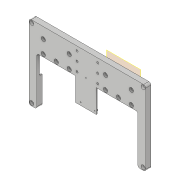
# Autodesk Inventor part: 10_Baseplate
Saved by Autodesk Inventor 2019 (Build 230136000, 136)
## iProperties
Created: 2019-05-14
Part Number: 10_Baseplate
Material: Generic
Document SubType Name: Modeling
Designer: diederichbenedict
Density: 1 g/cm^3
Appearance: Default
Author: diederichbenedict
Autodesk Inventor part; units mm, degrees
ref_plane "YZ Plane" through (0, 0, 0) normal (1, 0, 0) x (0, 1, 0)
ref_plane "XZ Plane" through (0, 0, 0) normal (0, 1, 0) x (-1, 0, 0)
ref_plane "XY Plane" through (0, 0, 0) normal (0, 0, 1) x (1, 0, 0)
ref_plane "Work Plane1" through (0, 0, 0) normal (0, 0, 1) x (1, 0, 0)
sketch "Sketch1" plane through (0, 0, 0) normal (0, 0, 1) x (1, 0, 0)
  circle A0 centre (0, 25) radius 1.95 construction
  circle A1 centre (-25, 0) radius 1.95 projected
  circle A2 centre (-25, -25) radius 1.95 projected
  circle A3 centre (25, 25) radius 1.95 construction
  circle A4 centre (25, -25) radius 1.95 projected
  circle A5 centre (-25, 25) radius 1.95 construction
  circle A6 centre (25, 0) radius 1.95 projected
  circle A7 centre (0, -25) radius 1.95 projected
  line L0 (-28, 30) -> (-30, 28) construction
  line L1 (-30, 28) -> (-30, -28) construction
  line L2 (-30, -28) -> (-28, -30) construction
  line L3 (-28, -30) -> (28, -30) construction
  line L4 (28, -30) -> (30, -28) construction
  line L5 (30, -28) -> (30, 28) construction
  line L6 (30, 28) -> (28, 30) construction
  line L7 (28, 30) -> (-28, 30) construction
  circle A8 centre (-145, 0) radius 1.95 projected
  circle A9 centre (-120, -25) radius 1.95 projected
  circle A10 centre (-95, -25) radius 1.95 projected
  circle A11 centre (-145, 25) radius 1.95 construction
  circle A12 centre (-95, 25) radius 1.95 construction
  circle A13 centre (-145, -25) radius 1.95 projected
  circle A14 centre (-120, 25) radius 1.95 construction
  circle A15 centre (-95, 0) radius 1.95 projected
  line L8 (-150, -28) -> (-148, -30) construction
  line L9 (-148, -30) -> (-92, -30) construction
  line L10 (-92, -30) -> (-90, -28) construction
  line L11 (-90, -28) -> (-90, 28) construction
  line L12 (-90, 28) -> (-92, 30) construction
  line L13 (-92, 30) -> (-148, 30) construction
  line L14 (-148, 30) -> (-150, 28) construction
  line L15 (-150, 28) -> (-150, -28) construction
  circle A16 centre (-167.5, -118) radius 1.95 projected
  circle A17 centre (47.5, -118) radius 1.95 construction
  circle A18 centre (47.5, 16) radius 1.95 projected
  circle A19 centre (-167.5, 16) radius 1.95 projected
  line L16 (52.5, -123) -> (-172.5, -123) construction
  line L17 (-172.5, -123) -> (-172.5, 21) construction
  line L18 (-172.5, 21) -> (52.5, 21) construction
  line L19 (52.5, 21) -> (52.5, -123) construction
  line L20 (52.5, -123) -> (37.5, -123) construction
  line L21 (37.5, -123) -> (37.5, 21) construction
  line L22 (37.5, 21) -> (52.5, 21) construction
  line L23 (52.5, 21) -> (52.5, -123) construction
  line L24 (-172.5, -123) -> (-157.5, -123) construction
  line L25 (-157.5, -123) -> (-157.5, 21) construction
  line L26 (-157.5, 21) -> (-172.5, 21) construction
  line L27 (-172.5, 21) -> (-172.5, -123) construction
  line L28 (-30, -30) -> (37.5, -30) construction
  line L29 (37.5, -30) -> (37.5, 21) construction
  line L30 (37.5, 21) -> (-30, 21) construction
  line L31 (-30, 21) -> (-30, -30) construction
  line L32 (-157.5, 21) -> (-90, 21) construction
  line L33 (-90, 21) -> (-90, -30) construction
  line L34 (-90, -30) -> (-157.5, -30) construction
  line L35 (-157.5, -30) -> (-157.5, 21) construction
  circle A20 centre (47.5, -118) radius 1.95
  line L36 (52.5, 21) -> (-172.5, 21)
  line L37 (-172.5, 21) -> (-172.5, -30)
  line L38 (-172.5, -30) -> (52.5, -30)
  line L39 (52.5, -30) -> (52.5, 21)
  line L40 (-172.5, -123) -> (-157.5, -123)
  line L41 (-157.5, -123) -> (-157.5, -30)
  line L42 (-157.5, -30) -> (-172.5, -30)
  line L43 (-172.5, -30) -> (-172.5, -123)
  line L44 (52.5, -123) -> (37.5, -123)
  line L45 (37.5, -123) -> (37.5, -30)
  line L46 (37.5, -30) -> (52.5, -30)
  line L47 (52.5, -30) -> (52.5, -123)
  line L48 (-80, 13) -> (-40, 13) construction
  line L49 (-40, 13) -> (-40, -22) construction
  line L50 (-40, -22) -> (-80, -22) construction
  line L51 (-80, -22) -> (-80, 13) construction
  line L52 (-80, 13) -> (-40, -22) construction
  line L53 (-40, 13) -> (-80, -22) construction
  circle A21 centre (-80, -4.5) radius 1.95
  circle A22 centre (-80, 13) radius 1.95
  circle A23 centre (-80, -22) radius 1.95
  circle A24 centre (-40, -22) radius 1.95
  circle A25 centre (-40, 13) radius 1.95
  circle A26 centre (-40, -4.5) radius 1.95
  point P0 (0, 0)
  point P1 (-60, -4.5)
  dimension "d0" = 5
  dimension "d1" = 5
  dimension "d2" = 5
  dimension "d3" = 5
  dimension "d4" = 15
  dimension "d5" = 15
  dimension "d33" = 40
  dimension "d34" = 35
  dimension "d35" = 17.5
  dimension "d36" = 17.5
  dimension "d37" = 3.9
  dimension "d38" = 3.9
  dimension "d39" = 3.9
  dimension "d40" = 3.9
  dimension "d41" = 3.9
  dimension "d42" = 3.9
  constraints: 76 end point, 18 parallel, 9 horizontal, 9 perpendicular, 7 centre point, 7 coincident, 4 midpoint, 4 point on line, 1 concentric
  measures "d0" distance from line of L19 A17.centre
  measures "d1" distance from line of A17.centre L16
  measures "d2" distance from line of A16.centre L17
  measures "d3" distance from line of A19.centre L18
  measures "d4" distance of L21.end L22.end
  measures "d5" distance of L26.end L25.end
  measures "d33" distance of L49.end L50.end
  measures "d34" distance of L48.end L49.end
  measures "d35" distance from line of point (-80, -4.5) L50
  measures "d36" distance from line of L50 point (-40, -4.5)
  measures "d37" diameter of A21
  measures "d38" diameter of A22
  measures "d39" diameter of A23
  measures "d40" diameter of A24
  measures "d41" diameter of A25
  measures "d42" diameter of A26
extrude "Extrusion1" add sketch "Sketch1" along normal blind 10
ref_plane "Work Plane2" through (-76.1, -69.7723, 8.1376) normal (0, -1, 0) x (-1, 0, 0)
ref_plane "Work Plane3" through (-64.05, -74.8223, 4.8376) normal (0, 1, 0) x (0, 0, 1)
sketch "Sketch2" plane through (-76.1, -69.7723, 8.1376) normal (0, -1, 0) x (-1, 0, 0)
  line L0 (6.9, 4.3) -> (-1.2981, 4.3) construction
  line L1 (-1.2981, 4.3) -> (-1.2981, 3.3) construction
  line L2 (-1.2981, 3.3) -> (0, 3.3) construction
  line L3 (0, 2.5) -> (0, 3.3) construction
  line L4 (0, 2.5) -> (-1.65, 2.5) construction
  line L5 (-1.65, 0) -> (-1.65, 2.5) construction
  line L6 (6.9, 0) -> (-1.65, 0) construction
  line L7 (6.9, 0) -> (6.9, 4.3) construction
  line L8 (-32.1, 2.3) -> (-32.1, 4.3) construction
  line L9 (-32.1, 4.3) -> (-33.3, 4.3) construction
  line L10 (-33.3, 0) -> (-33.3, 4.3) construction
  line L11 (-33.3, 0) -> (-28.35, 0) construction
  line L12 (-28.35, 0) -> (-28.35, 2.3) construction
  line L13 (-28.35, 2.3) -> (-32.1, 2.3) construction
  line L14 (81.4, -1.8624) -> (-113.6, -1.8624) construction
  line L15 (-33.3, 0) -> (6.9, 0)
  line L16 (6.9, 0) -> (6.9, -1.8624)
  line L17 (6.9, -1.8624) -> (-33.3, -1.8624)
  line L18 (-33.3, -1.8624) -> (-33.3, 0)
  point P0 (-76.1, 8.1376)
  constraints: 8 end point, 2 parallel, 1 horizontal, 1 perpendicular, 1 point on line
extrude "Extrusion2" add sketch "Sketch2" along normal up to surface (44.8223 mm away) from surface at -39.7723
sketch "Sketch3" plane through (-42.8, -69.7723, 8.1376) normal (0, 0, -1) x (-1, 0, 0)
  line L0 (0, 39.7723) -> (40.2, 39.7723) projected
  line L1 (0, 39.7723) -> (0, -5.05) projected
  line L2 (40.2, -5.05) -> (40.2, 39.7723) projected
  line L3 (114.7, 39.7723) -> (40.2, 39.7723) projected
  arc A0 (40.2, 39.7723) -> (0, 39.7723) centre (20.1, 30.1966) ccw
  line L4 (40.2, -5.05) -> (0, -5.05) projected
  point P0 (-42.8, 69.7723)
  constraints: 2 point on circle, 1 centre point
extrude "Extrusion3" cut sketch "Sketch3" along normal up to surface (8.1376 mm away) contours A0 L0
sketch "Sketch4" plane through (-42.8, -74.8223, 8.1376) normal (0, 0, -1) x (-1, 0, 0)
  circle A0 centre (3.3, 4.4309) radius 0.9 projected
  circle A1 centre (20, 51.15) radius 0.9 projected
  circle A2 centre (30.3, 5.3) radius 0.9 projected
  point P0 (-42.8, 74.8223)
extrude "Extrusion4" cut sketch "Sketch4" against normal through all
sketch "Sketch5" plane through (-42.8, -74.8223, 8.1376) normal (0, 0, -1) x (-1, 0, 0)
  circle A0 centre (20, 51.15) radius 0.9 projected
  circle A1 centre (3.3, 4.4309) radius 0.9 projected
  circle A2 centre (30.3, 5.3) radius 0.9 projected
  circle A3 centre (20, 51.15) radius 2.1
  circle A4 centre (3.3, 4.4309) radius 2.1
  circle A5 centre (30.3, 5.3) radius 2.1
  point P0 (-42.8, 74.8223)
  dimension "d14" = 1.2
  dimension "d15" = 1.2
  dimension "d16" = 1.2
  constraints: 3 centre point
  measures "d14" radial gap between concentric circles of A0 A3
  measures "d15" radial gap between concentric circles of A1 A4
  measures "d16" radial gap between concentric circles of A2 A5
ref_plane "Work Plane4" through (-51.8, -75.6302, 5.8376) normal (0, 0, 1) x (1, 0, 0)
extrude "Extrusion5" add sketch "Sketch5" along normal up to surface (2.3 mm away)
sketch "Sketch6" plane through (-62.8, -23.6723, 5.8376) normal (0, 0, -1) x (-1, 0, 0)
  circle A0 centre (0, 0) radius 2.1 projected
  circle A1 centre (0, 0) radius 0.9 projected
  point P0 (-62.8, 23.6723)
ref_plane "Work Plane5" through (-72.8, -36.4723, 4.6376) normal (0, 0, 1) x (1, 0, 0)
extrude "Extrusion6" add sketch "Sketch6" along normal up to surface (1.2 mm away)
fillet "Fillet1" radius 4 8 edges at (37.5, -123, 5) (52.5, -123, 5) (37.5, -30, 5) (-172.5, -123, 5) (-157.5, -123, 5) (-157.5, -30, 5) (-172.5, 21, 5) (52.5, 21, 5)
sketch "Sketch7" plane through (0, 0, 10) normal (0, 0, 1) x (1, 0, 0)
  arc A0 (52.5, 17) -> (48.5, 21) centre (48.5, 17) ccw projected
  line L0 (48.5, 21) -> (-168.5, 21) projected
  arc A1 (-168.5, 21) -> (-172.5, 17) centre (-168.5, 17) ccw projected
  line L1 (-172.5, 17) -> (-172.5, -119) projected
  arc A2 (-172.5, -119) -> (-168.5, -123) centre (-168.5, -119) ccw projected
  line L2 (-168.5, -123) -> (-161.5, -123) projected
  arc A3 (-161.5, -123) -> (-157.5, -119) centre (-161.5, -119) ccw projected
  line L3 (-157.5, -119) -> (-157.5, -34) projected
  arc A4 (-153.5, -30) -> (-157.5, -34) centre (-153.5, -34) ccw projected
  line L4 (-153.5, -30) -> (-83, -30) projected
  line L5 (-83, -74.8223) -> (-83, -30) projected
  line L6 (-42.8, -74.8223) -> (-83, -74.8223) projected
  line L7 (-42.8, -74.8223) -> (-42.8, -30) projected
  line L8 (-42.8, -30) -> (33.5, -30) projected
  arc A5 (37.5, -34) -> (33.5, -30) centre (33.5, -34) ccw projected
  line L9 (37.5, -34) -> (37.5, -119) projected
  arc A6 (37.5, -119) -> (41.5, -123) centre (41.5, -119) ccw projected
  line L10 (41.5, -123) -> (48.5, -123) projected
  arc A7 (48.5, -123) -> (52.5, -119) centre (48.5, -119) ccw projected
  line L11 (52.5, -119) -> (52.5, 17) projected
  circle A8 centre (-62.8, -23.6723) radius 0.9 projected
  circle A9 centre (-46.1, -70.3914) radius 0.9 projected
  circle A10 centre (-73.1, -69.5223) radius 0.9 projected
  circle A11 centre (-167.5, 16) radius 1.95 projected
  circle A12 centre (47.5, 16) radius 1.95 projected
  circle A13 centre (-95, 0) radius 1.95 projected
  circle A14 centre (-145, -25) radius 1.95 projected
  circle A15 centre (-95, -25) radius 1.95 projected
  circle A16 centre (-120, -25) radius 1.95 projected
  circle A17 centre (-145, 0) radius 1.95 projected
  circle A18 centre (0, -25) radius 1.95 projected
  circle A19 centre (25, 0) radius 1.95 projected
  circle A20 centre (25, -25) radius 1.95 projected
  circle A21 centre (-25, -25) radius 1.95 projected
  circle A22 centre (-25, 0) radius 1.95 projected
  circle A23 centre (-167.5, -118) radius 1.95 projected
  circle A24 centre (47.5, -118) radius 1.95 projected
  circle A25 centre (-40, -4.5) radius 1.95 projected
  circle A26 centre (-40, 13) radius 1.95 projected
  circle A27 centre (-40, 13) radius 1.95 projected
  circle A28 centre (-40, -22) radius 1.95 projected
  circle A29 centre (-40, -22) radius 1.95 projected
  circle A30 centre (-80, -22) radius 1.95 projected
  circle A31 centre (-80, -4.5) radius 1.95 projected
  circle A32 centre (-80, -4.5) radius 1.95 projected
  circle A33 centre (-80, 13) radius 1.95 projected
  circle A34 centre (-80, 13) radius 1.95 projected
  point P0 (0, 0)
hole "Hole1" at (47.5, 16, 10) at (25, 0, 10) at (25, -25, 10) at (0, -25, 10) at (-25, -25, 10) at (-25, 0, 10) at (-95, -25, 10) at (-95, 0, 10) at (-120, -25, 10) at (-145, -25, 10) at (-145, 0, 10) at (-167.5, 16, 10) at (-167.5, -118, 10) at (47.5, -118, 10) direction (0, 0, -1) diameter 2 depth 10 tip angle 118 counterbore diameter 8 counterbore depth 4
shell "Shell1" thickness 2 removed faces 1 at (-167.5, -45.3333, 0)
sketch "Sketch8" plane through (39.5, -119, 8) normal (1, 0, 0) x (0, 0, -1)
  line L0 (8, 0) -> (8, 85) projected
  line L1 (8, 84.9782) -> (5.0703, 84.9782)
  line L2 (3.0703, 82.9782) -> (3.0703, 51.1801)
  line L3 (5.0703, 49.1801) -> (8, 49.1801)
  line L4 (8, 49.1801) -> (8, 84.9782)
  arc A0 (5.0703, 84.9782) -> (3.0703, 82.9782) centre (5.0703, 82.9782) ccw
  arc A1 (3.0703, 51.1801) -> (5.0703, 49.1801) centre (5.0703, 51.1801) ccw
  point P0 (8, 119)
  dimension "d30" = 2
  constraints: 8 end point, 4 point on circle, 4 tangent, 2 centre point, 2 parallel, 1 equal radius, 1 horizontal, 1 perpendicular, 1 point on line
  measures "d30" radius of A0
extrude "Extrusion7" cut sketch "Sketch8" against normal up to surface (199 mm away)
body "Solid1"
